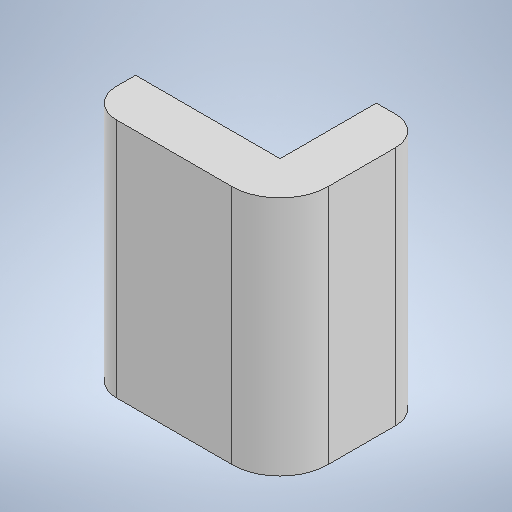
# Autodesk Inventor part: F4-freeze
Saved by Autodesk Inventor 2025.2 (Build 292293000, 293)
## iProperties
Created: 2025-11-18
Part Number: F4-freeze
Material: 일반
Document SubType Name: Modeling
Designer: RunGeun
Density: 1 g/cm^3
Appearance: 기본값
Author: RunGeun
Autodesk Inventor part; units mm, degrees
ref_plane "YZ Plane" through (0, 0, 0) normal (1, 0, 0) x (0, 1, 0)
ref_plane "XZ Plane" through (0, 0, 0) normal (0, 1, 0) x (-1, 0, 0)
ref_plane "XY Plane" through (0, 0, 0) normal (0, 0, 1) x (1, 0, 0)
sketch "스케치1" plane through (0, 0, 0) normal (0, 1, 0) x (-1, 0, 0)
  line L0 (0, 0) -> (2, 0)
  line L1 (2, 0) -> (2, -6)
  line L2 (2, -6) -> (0, -6)
  line L3 (0, -6) -> (0, 0)
  line L4 (2, -2) -> (8, -2)
  line L5 (8, -2) -> (8, 0)
  line L6 (8, 0) -> (2, 0)
  line L7 (2, 0) -> (2, -2)
  point P0 (1, -6)
  dimension "d0" = 6
  dimension "d1" = 4
  dimension "d2" = 2
  dimension "d3" = 2
  constraints: 16 end point, 4 parallel, 2 horizontal, 2 perpendicular, 2 point on line, 1 midpoint
  measures "d0" distance of L4.start L4.end
  measures "d1" distance from line of L4 point (1, -6)
  measures "d2" distance of L1.end L2.end
  measures "d3" distance of L4.end L5.end
extrude "돌출1" add sketch "스케치1" along normal blind 10
fillet "모깎기1" radius 2 1 edges at (0, 5, 0)
fillet "모깎기2" radius 1.2 2 edges at (0, 5, -6) (-8, 5, 0)
